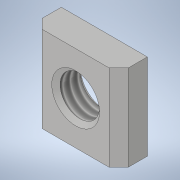
# Autodesk Inventor part: T-Nut Block M5  Threads
Saved by Autodesk Inventor 2022 (Build 260153000, 153)
## iProperties
Category: PARTsolutions
Company: 8020
Created: 2022-09-20
Part Number: T-Nut Block M5  Threads
Material: Generic
Catalog Web Link: www.cadenas.de
Description: 14159, 14122, 14124, 14126, 14127, 14128, 14129, 14130, 14131_m-Slide-In Economy T-Nuts
Vendor: 8020
Document SubType Name: Modeling
Designer: psAdmin
Manufacturer: 8020
Mass: 0.191128 g
Surface Area: 2.63473 cm^2
Volume: 0.191128 cm^3
Density: 1 g/cm^3
Appearance: PSOLRGB-175-175-175
PSOL_IDENT_0: {$CADENAS_DATA/23d-libs/8020/metric/fastening_options/14159_m.prj},209 {VTYP=3D},{NB=14122_m},{LINA=
PSOL_IDENT_1: 14122},{NN=14159, 14122, 14124, 14126, 14127, 14128, 14129, 14130, 14131_m},{DATE=31.07.2020 09:21:2
PSOL_IDENT_2: 6},{GEOMDATE=20.06.2019 14:19:00},{VERSION=},{LINEID=20},{WBVAR=},{WBNUMERIC=}  {NB=14122_m},{LINA=1
PSOL_IDENT_3: 4122},{KT=DUMMY},{PN=14122},{MAT=Steel},{FIN=Zinc-Plated},{A=M5},{A1=5},{B=9.00},{C=9.00},{D=3.00},{
PSOL_IDENT_4: CC=5-20}
NB: 14122_m
NN: 14159, 14122, 14124, 14126, 14127, 14128, 14129, 14130, 14131_m
NT: Slide-In Economy T-Nuts
NBSYN: $PN._m
LINA: 14122
CATALOG: 80/20
PN: 14122
MAT: Steel
FIN: Zinc-Plated
A: M5
B: 9
C: 9
D: 3
CC: 5-20
SUPPLIER: 8020
ARTICLENO: 14122_m
BOMINFO: 14122
CREATOR: CADENAS GmbH
Title: 14122
Author: Cadenas PARTsolutions
Comments: Slide-In Economy T-Nuts
Autodesk Inventor part; units mm, degrees
ref_plane "YZ Plane" through (0, 0, 0) normal (1, 0, 0) x (0, 1, 0)
ref_plane "XZ Plane" through (0, 0, 0) normal (0, 1, 0) x (-1, 0, 0)
ref_plane "XY Plane" through (0, 0, 0) normal (0, 0, 1) x (1, 0, 0)
sketch "Sketch_1" plane through (0, 0, 0) normal (0, 0, 1) x (1, 0, 0)
  line L0 (-4.5, 4.5) -> (-4.5, -4.5)
  line L1 (-4.5, -4.5) -> (4.5, -4.5)
  line L2 (4.5, -4.5) -> (4.5, 4.5)
  line L3 (4.5, 4.5) -> (-4.5, 4.5)
  constraints: 8 end point
extrude "Extrusion1" add sketch "Sketch_1" along normal mid plane 3
sketch "Sketch_2" plane through (0, 0, 0) normal (1, 0, 0) x (0, 1, 0)
  line L0 (0, -1.5) -> (0, 1.5)
  line L1 (0, 1.5) -> (2.5, 1.5)
  line L2 (2.5, 1.5) -> (2.067, 1.067)
  line L3 (2.067, 1.067) -> (2.067, -1.067)
  line L4 (2.067, -1.067) -> (2.5, -1.5)
  line L5 (2.5, -1.5) -> (0, -1.5)
  line L6 (0, -1.5) -> (0, 1.5)
  constraints: 14 end point
revolve "Revolution1" cut sketch "Sketch_2" angle 360 about axis through (0, 0, -1.5) along (0, 0, -1)
thread "Thread1" size "M5x0.8" class "6H" standard "ISO Metric profile" full length
sketch "Sketch_3" plane through (0, 0, 0) normal (0, 1, 0) x (-1, 0, 0)
  line L0 (4.5, 0.5) -> (4.5, 2.5)
  line L1 (4.5, 2.5) -> (-4.5, 2.5)
  line L2 (-4.5, 2.5) -> (-4.5, 0.5)
  line L3 (-4.5, 0.5) -> (-3.5, 1.5)
  line L4 (-3.5, 1.5) -> (3.5, 1.5)
  line L5 (3.5, 1.5) -> (4.5, 0.5)
  constraints: 12 end point
extrude "Extrusion2" cut sketch "Sketch_3" along normal mid plane 18
ref_plane "Work Plane1" through (-4.5, 0, -1.5) normal (0, 1, 0) x (1, 0, 0)
body "Solid1"
